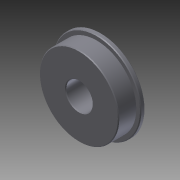
# Autodesk Inventor part: fr-6-zz (1.125 OD Version)
Saved by Autodesk Inventor 2014 SP1 (Build 180222100, 222)
## iProperties
Created: 2012-02-08
Part Number: fr-6-zz (1.125 OD Version)
Material: Steel
Document SubType Name: Modeling
Designer: Moses
Density: 7.85 g/cm^3
Mass: 37.491 g
Surface Area: 23.5952 cm^2
Volume: 4.77593 cm^3
Appearance: Steel
Author: Moses
Autodesk Inventor part; units mm, degrees
ref_plane "YZ Plane" through (0, 0, 0) normal (1, 0, 0) x (0, 1, 0)
ref_plane "XZ Plane" through (0, 0, 0) normal (0, 1, 0) x (-1, 0, 0)
ref_plane "XY Plane" through (0, 0, 0) normal (0, 0, 1) x (1, 0, 0)
sketch "Sketch1" plane through (0, 0, 0) normal (0, 0, 1) x (1, 0, 0)
  circle A0 centre (0, 0) radius 14.2875
  circle A1 centre (0, 0) radius 4.7625
  circle A2 centre (0, 0) radius 15.875
  dimension "d0" = 28.575
  dimension "d1" = 9.525
  dimension "d2" = 31.75
  constraints: 3 centre point, 3 coincident
  measures "d0" diameter of A0
  measures "d1" diameter of A1
  measures "d2" diameter of A2
extrude "Extrusion1" add sketch "Sketch1" along normal blind 6.3754 contours A0
extrude "Extrusion2" add sketch "Sketch1" against normal blind 1.6002 contours A0 | A2
chamfer "Chamfer1" distance 0.254 angle 45 5 edges at (-14.2875, 0, 6.3754) (-15.875, 0, 0) (-15.875, 0, -1.6002) (-4.7625, 0, 6.3754) (-4.7625, 0, -1.6002)
body "Solid1"
